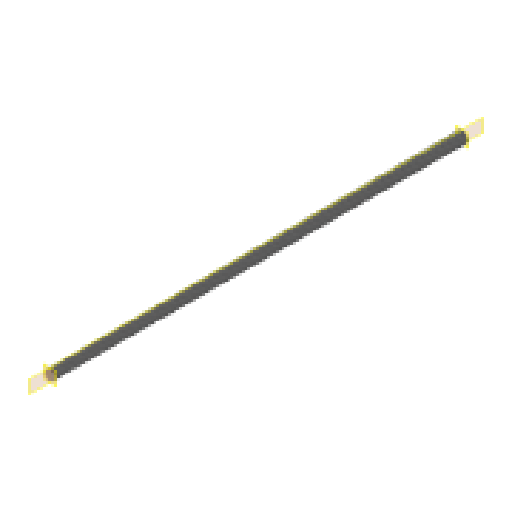
# Autodesk Inventor part: Fuselage JF
Saved by Autodesk Inventor 2025.1 (Build 291241000, 241)
## iProperties
Created: 2025-01-07
Part Number: Fuselage JF
Material: Generic
Document SubType Name: Modeling
Designer: alptl
Density: 1 g/cm^3
Appearance: Default
Author: alptl
Autodesk Inventor part; units mm, degrees
ref_plane "XZ Plane" through (0, 0, 0) normal (0, 1, 0) x (-1, 0, 0)
sketch "Sketch1" plane through (0, 0, 0) normal (0, 0, 1) x (1, 0, 0)
  circle A0 centre (0, 0) radius 20
  dimension "d0" = 40
  constraints: 1 centre point, 1 coincident
  measures "d0" diameter of A0
sketch "Sketch2" plane through (0, 0, 0) normal (1, 0, 0) x (0, 1, 0)
  line L0 (0, 0) -> (0, 1400)
  point P0 (0, 350)
  point P1 (0, 450)
  point P2 (0, 1240)
  point P3 (0, 1340)
  dimension "d1" = 1400
  constraints: 4 point on line, 2 end point, 1 vertical
  measures "d1" distance of L0.start L0.end
ref_plane "Work Plane1" through (0, 0, 1400) normal (0, 0, 1) x (1, 0, 0)
sketch "Sketch3" plane through (0, 0, 1400) normal (0, 0, 1) x (1, 0, 0)
  circle A0 centre (0, 0) radius 17.665
  dimension "d4" = 35.33
  constraints: 1 centre point, 1 coincident
  measures "d4" diameter of A0
loft "Loft1" add profiles "Sketch1", "Sketch3"
hole "Hole1" at (0, 0, 350) at (0, 0, 450) at (0, 0, 1240) at (0, 0, 1340) direction (-1, 0, 0) diameter 4.8 depth 21.567 start extended yes
body "Solid1"
